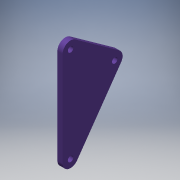
# Autodesk Inventor part: carriage plate
Saved by Autodesk Inventor 2017 SP1 (Build 210196100, 196)
## iProperties
Created: 2018-01-19
Part Number: carriage plate
Material: Aluminum 6061
Document SubType Name: Modeling
Designer: Ben
Density: 2.7 g/cm^3
Appearance: Violet
Mass: 99.9601 g
Surface Area: 141.524 cm^2
Volume: 37.0222 cm^3
Author: Ben
Autodesk Inventor part; units mm, degrees
ref_plane "YZ Plane" through (0, 0, 0) normal (1, 0, 0) x (0, 1, 0)
ref_plane "XZ Plane" through (0, 0, 0) normal (0, 1, 0) x (-1, 0, 0)
ref_plane "XY Plane" through (0, 0, 0) normal (0, 0, 1) x (1, 0, 0)
sketch "Sketch1" plane through (0, 0, 0) normal (1, 0, 0) x (0, 1, 0)
  line L0 (-420.7488, 12.7) -> (420.7488, 12.7) construction
  line L1 (420.7488, 12.7) -> (420.7488, -12.7)
  line L2 (420.7488, -12.7) -> (-420.7488, -12.7) construction
  line L3 (-420.7488, -12.7) -> (-420.7488, 12.7)
  line L4 (0, 0) -> (0, -26.6192) construction
  circle A0 centre (0, -26.6192) radius 3.302
  line L5 (420.7488, 0) -> (-420.7488, 0) construction
  circle A1 centre (38.1, 26.6192) radius 3.302
  circle A2 centre (-76.2, 26.6192) radius 3.302
  line L6 (38.1, 26.6192) -> (-76.2, 26.6192) construction
  line L7 (0, 0) -> (0, 26.6192) construction
  circle A3 centre (0, -26.6192) radius 15.875 construction
  circle A4 centre (38.1, 26.6192) radius 15.875 construction
  circle A5 centre (-76.2, 26.6192) radius 15.875 construction
  line L8 (0, -26.6192) -> (-76.2, 26.6192) construction
  arc A6 (45.8458, 21.0759) -> (38.1, 36.1442) centre (38.1, 26.6192) ccw
  arc A7 (-76.2, 36.1442) -> (-81.6552, 18.8111) centre (-76.2, 26.6192) ccw
  arc A8 (-5.4552, -34.4273) -> (7.7458, -32.1625) centre (0, -26.6192) ccw
  line L9 (38.1, 36.1442) -> (-76.2, 36.1442)
  line L10 (45.8458, 21.0759) -> (7.7458, -32.1625)
  line L11 (-5.4552, -34.4273) -> (-81.6552, 18.8111)
  dimension "d0" = 25.4
  dimension "d1" = 6.604
  dimension "d2" = 13.9192
  dimension "d3" = 31.75
  dimension "d4" = 38.1
  dimension "d5" = 76.2
  dimension "d6" = 9.525
  constraints: 24 end point, 9 centre point, 8 coincident, 6 equal radius, 6 point on circle, 5 tangent, 3 horizontal, 3 midpoint, 2 parallel, 2 perpendicular, 1 collinear, 1 point on line, 1 vertical
  measures "d0" distance of L0.end L1.end
  measures "d1" diameter of A0
  measures "d2" distance from line of L2 L4.end
  measures "d3" diameter of A3
  measures "d4" horizontal distance of L6.start L4.end
  measures "d5" distance from line of A2.centre L7
  measures "d6" radius of A6
extrude "Extrusion1" add sketch "Sketch1" along normal blind 6.35
body "Solid1"
